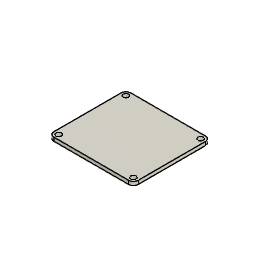
Power Mount Panel Compact - BLANK (Autodesk Fusion 360 design; units mm, degrees)
Autodesk Fusion 360 part; units mm, degrees
sketch "Sketch1" plane through (0, 0, 0) normal (0, 0, 1) x (1, 0, 0)
  line L0 (-22.8127, 21.0938) -> (39.6873, 21.0938) construction
  line L1 (39.6873, 21.0938) -> (39.6873, -35.1562) construction
  line L2 (39.6873, -35.1562) -> (-22.8127, -35.1562) construction
  line L3 (-22.8127, -35.1562) -> (-22.8127, 21.0938) construction
  circle A0 centre (-22.8127, 21.0938) radius 2.25
  circle A1 centre (39.6873, 21.0938) radius 2.25
  circle A2 centre (39.6873, -35.1562) radius 2.25
  circle A3 centre (-22.8127, -35.1562) radius 2.25
  circle A4 centre (-22.8127, 21.0938) radius 4
  circle A5 centre (39.6873, 21.0938) radius 4
  circle A6 centre (-22.8127, -35.1562) radius 4
  circle A7 centre (39.6873, -35.1562) radius 4
  line L4 (-26.8127, 21.0938) -> (-26.8127, -35.1562)
  line L5 (-22.8127, 25.0938) -> (39.6873, 25.0938)
  line L6 (43.6873, 21.0938) -> (43.6873, -35.1562)
  line L7 (39.6873, -39.1562) -> (-22.8127, -39.1562)
  dimension "d1" = 62.5
  dimension "d2" = 56.25
  dimension "d3" = 4.5
  dimension "d4" = 4.5
  dimension "d5" = 4.5
  dimension "d6" = 4.5
  dimension "d7" = 8
  dimension "d8" = 8
  dimension "d9" = 8
  dimension "d10" = 8
  constraint horizontal L0
  constraint vertical L1
  constraint horizontal L2
  constraint vertical L3
  constraint coincident L0.start L3.end
  constraint coincident L0.end L1.start
  constraint coincident L1.end L2.start
  constraint coincident L2.end L3.start
  constraint concentric A0 A4
  constraint concentric A1 A5
  constraint concentric A3 A6
  constraint concentric A2 A7
  constraint coincident A4 L4.start
  constraint coincident A6 L4.end
  constraint tangent A6 L4
  constraint tangent A4 L4
  constraint coincident A4 L5.start
  constraint coincident A5 L5.end
  constraint tangent A5 L5
  constraint tangent A4 L5
  constraint coincident A5 L6.start
  constraint coincident A7 L6.end
  constraint tangent A7 L6
  constraint tangent A5 L6
  constraint coincident A7 L7.start
  constraint coincident A6 L7.end
  constraint tangent A6 L7
  constraint tangent A7 L7
  measures "d1" distance of L0.start L0.end
  measures "d2" distance of L0.end L1.end
  measures "d3" diameter of A0
  measures "d4" diameter of A1
  measures "d5" diameter of A2
  measures "d6" diameter of A3
  measures "d7" diameter of A4
  measures "d8" diameter of A5
  measures "d9" diameter of A6
  measures "d10" diameter of A7
extrude "Extrude1" add sketch "Sketch1" along normal blind 3
equation "d4 = d3"
equation "d5 = d3"
equation "d6 = d3"
equation "d8 = d7"
equation "d9 = d7"
equation "d10 = d7"
